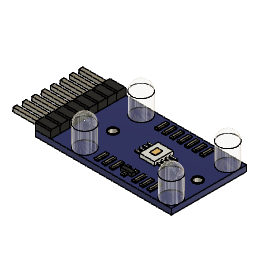
TCS3200_colour_sensor (Autodesk Fusion 360 design; units mm, degrees)
Autodesk Fusion 360 part; units mm, degrees
sketch "Circuitboard shape" plane through (0, 0, 0) normal (0, 0, 1) x (1, 0, 0)
  line L0 (0, 0) -> (36, 0)
  line L1 (36, 0) -> (36, 20)
  line L2 (36, 20) -> (0, 20)
  line L3 (0, 20) -> (0, 0)
  dimension "d1" = 20
  dimension "d2" = 36
  constraint horizontal L0
  constraint vertical L1
  constraint horizontal L2
  constraint vertical L3
  constraint coincident L0.start L3.end
  measures "d1" distance of L0.start L2.end
  measures "d2" distance of L0.start L0.end
extrude "Extrude1" add sketch "Circuitboard shape" along normal blind 1.5 makes body 1
sketch "Black Pin Connectors" plane through (0, 0, 1.5) normal (0, 0, 1) x (-1, 0, 0)
  line L0 (0, -20) -> (0, 0)
  line L1 (0, 0) -> (-36, 0)
  line L2 (-36, 0) -> (-36, -20)
  line L3 (-36, -20) -> (0, -20)
  line L4 (0, -20) -> (-4, -20)
  line L5 (-4, -20) -> (-4, -17.5)
  line L6 (-4, -17.5) -> (0, -17.5)
  line L7 (0, -17.5) -> (0, -20)
  line L8 (-4, -17.5) -> (0, -17.5)
  line L9 (0, -17.5) -> (0, -15)
  line L10 (0, -15) -> (-4, -15)
  line L11 (-4, -15) -> (-4, -17.5)
  line L12 (-4, -15) -> (0, -15)
  line L13 (0, -15) -> (0, -12.5)
  line L14 (0, -12.5) -> (-4, -12.5)
  line L15 (-4, -12.5) -> (-4, -15)
  line L16 (-4, -12.5) -> (0, -12.5)
  line L17 (0, -12.5) -> (0, -10)
  line L18 (0, -10) -> (-4, -10)
  line L19 (-4, -10) -> (-4, -12.5)
  line L20 (-4, -10) -> (0, -10)
  line L21 (0, -10) -> (0, -7.5)
  line L22 (0, -7.5) -> (-4, -7.5)
  line L23 (-4, -7.5) -> (-4, -10)
  line L24 (-4, -7.5) -> (0, -7.5)
  line L25 (0, -7.5) -> (0, -5)
  line L26 (0, -5) -> (-4, -5)
  line L27 (-4, -5) -> (-4, -7.5)
  line L28 (-4, -5) -> (0, -5)
  line L29 (0, -5) -> (0, -2.5)
  line L30 (0, -2.5) -> (-4, -2.5)
  line L31 (-4, -2.5) -> (-4, -5)
  line L32 (-4, -2.5) -> (0, -2.5)
  line L33 (0, -2.5) -> (0, 0)
  line L34 (0, 0) -> (-4, 0)
  line L35 (-4, 0) -> (-4, -2.5)
  dimension "d5" = 2.5
  dimension "d6" = 2.5
  dimension "d7" = 2.5
  dimension "d8" = 2.5
  dimension "d9" = 2.5
  dimension "d10" = 2.5
  dimension "d11" = 2.5
  dimension "d12" = 2.5
  dimension "d13" = 4
  constraint horizontal L4
  constraint vertical L5
  constraint horizontal L6
  constraint vertical L7
  constraint coincident L0.start L3.end
  constraint horizontal L8
  constraint vertical L9
  constraint horizontal L10
  constraint vertical L11
  constraint coincident L0 L9.end
  constraint horizontal L12
  constraint vertical L13
  constraint horizontal L14
  constraint vertical L15
  constraint coincident L0 L13.end
  constraint horizontal L16
  constraint vertical L17
  constraint horizontal L18
  constraint vertical L19
  constraint coincident L0 L17.end
  constraint horizontal L20
  constraint vertical L21
  constraint horizontal L22
  constraint vertical L23
  constraint coincident L0 L21.end
  constraint horizontal L24
  constraint vertical L25
  constraint horizontal L26
  constraint vertical L27
  constraint coincident L0 L25.end
  constraint horizontal L28
  constraint vertical L29
  constraint horizontal L30
  constraint vertical L31
  constraint coincident L0 L29.end
  constraint horizontal L32
  constraint vertical L33
  constraint horizontal L34
  constraint vertical L35
  constraint coincident L0.end L1.start
  measures "d5" distance of L4.end L5.end
  measures "d6" distance of L5.end L10.end
  measures "d7" distance of L10.end L14.end
  measures "d8" distance of L14.end L18.end
  measures "d9" distance of L18.end L22.end
  measures "d10" distance of L22.end L26.end
  measures "d11" distance of L26.end L30.end
  measures "d12" distance of L30.end L34.end
  measures "d13" distance of L0.end L34.end
extrude "Extrude2" add sketch "Black Pin Connectors" along normal blind 2 separate body contours L0 L3 L4 L5 L6 L7 L8 | L0 L10 L12 L13 L14 L15 L16 | L0 L18 L20 L21 L22 L23 L24 | L0 L26 L28 L29 L30 L31 L32 makes body 2 at (1.3333, 14.1667, 1.5) makes body 3 at (1.3333, 9.1667, 1.5) makes body 4 at (1.3333, 19.1667, 1.5) makes body 5 at (2.6667, 3.3333, 1.5)
chamfer "Chamfer1" distance 0.3 angle 45 8 edges at (2, 10, 3.5) (2, 7.5, 3.5) (2, 15, 3.5) (2, 12.5, 3.5) (2, 20, 3.5) (2, 17.5, 3.5) (2, 5, 3.5) (2, 2.5, 3.5) on bodies 2 3 4 5
extrude "Extrude3" add sketch "Black Pin Connectors" along normal blind 2 separate body contours L0 L6 L8 L9 L10 L11 L12 | L0 L14 L16 L17 L18 L19 L20 | L0 L1 L30 L32 L33 L34 L35 | L0 L22 L24 L25 L26 L27 L28 makes body 6 at (1.3333, 11.6667, 1.5) makes body 7 at (1.3333, 6.6667, 1.5) makes body 8 at (1.3333, 16.6667, 1.5) makes body 9 at (2.6667, 0.8333, 1.5)
chamfer "Chamfer2" distance 0.3 angle 45 8 edges at (2, 2.5, 3.5) (2, 0, 3.5) (2, 12.5, 3.5) (2, 10, 3.5) (2, 7.5, 3.5) (2, 5, 3.5) (2, 17.5, 3.5) (2, 15, 3.5) on bodies 6 7 8 9
sketch "Pins" plane through (0, 0, 0) normal (-1, 0, 0) x (0, -1, 0)
  line L0 (-17.5, 3.2) -> (-17.8, 3.5)
  line L1 (-17.8, 3.5) -> (-19.7, 3.5)
  line L2 (-19.7, 3.5) -> (-20, 3.2)
  line L3 (-20, 3.2) -> (-20, 1.5)
  line L4 (-20, 1.5) -> (-17.5, 1.5)
  line L5 (-17.5, 1.5) -> (-17.5, 3.2)
  line L6 (-15, 3.2) -> (-15.3, 3.5)
  line L7 (-15.3, 3.5) -> (-17.2, 3.5)
  line L8 (-17.2, 3.5) -> (-17.5, 3.2)
  line L9 (-17.5, 3.2) -> (-17.5, 1.5)
  line L10 (-17.5, 1.5) -> (-15, 1.5)
  line L11 (-15, 1.5) -> (-15, 3.2)
  line L12 (-12.5, 3.2) -> (-12.8, 3.5)
  line L13 (-12.8, 3.5) -> (-14.7, 3.5)
  line L14 (-14.7, 3.5) -> (-15, 3.2)
  line L15 (-15, 3.2) -> (-15, 1.5)
  line L16 (-15, 1.5) -> (-12.5, 1.5)
  line L17 (-12.5, 1.5) -> (-12.5, 3.2)
  line L18 (-10, 3.2) -> (-10.3, 3.5)
  line L19 (-10.3, 3.5) -> (-12.2, 3.5)
  line L20 (-12.2, 3.5) -> (-12.5, 3.2)
  line L21 (-12.5, 3.2) -> (-12.5, 1.5)
  line L22 (-12.5, 1.5) -> (-10, 1.5)
  line L23 (-10, 1.5) -> (-10, 3.2)
  line L24 (-7.5, 3.2) -> (-7.8, 3.5)
  line L25 (-7.8, 3.5) -> (-9.7, 3.5)
  line L26 (-9.7, 3.5) -> (-10, 3.2)
  line L27 (-10, 3.2) -> (-10, 1.5)
  line L28 (-10, 1.5) -> (-7.5, 1.5)
  line L29 (-7.5, 1.5) -> (-7.5, 3.2)
  line L30 (-5, 3.2) -> (-5.3, 3.5)
  line L31 (-5.3, 3.5) -> (-7.2, 3.5)
  line L32 (-7.2, 3.5) -> (-7.5, 3.2)
  line L33 (-7.5, 3.2) -> (-7.5, 1.5)
  line L34 (-7.5, 1.5) -> (-5, 1.5)
  line L35 (-5, 1.5) -> (-5, 3.2)
  line L36 (-2.5, 3.2) -> (-2.8, 3.5)
  line L37 (-2.8, 3.5) -> (-4.7, 3.5)
  line L38 (-4.7, 3.5) -> (-5, 3.2)
  line L39 (-5, 3.2) -> (-5, 1.5)
  line L40 (-5, 1.5) -> (-2.5, 1.5)
  line L41 (-2.5, 1.5) -> (-2.5, 3.2)
  line L42 (0, 3.2) -> (-0.3, 3.5)
  line L43 (-0.3, 3.5) -> (-2.2, 3.5)
  line L44 (-2.2, 3.5) -> (-2.5, 3.2)
  line L45 (-2.5, 3.2) -> (-2.5, 1.5)
  line L46 (-2.5, 1.5) -> (0, 1.5)
  line L47 (0, 1.5) -> (0, 3.2)
  line L48 (-19.25, 3) -> (-18.25, 3)
  line L49 (-18.25, 3) -> (-18.25, 2)
  line L50 (-18.25, 2) -> (-19.25, 2)
  line L51 (-19.25, 2) -> (-19.25, 3)
  line L52 (-16.75, 3) -> (-15.75, 3)
  line L53 (-15.75, 3) -> (-15.75, 2)
  line L54 (-15.75, 2) -> (-16.75, 2)
  line L55 (-16.75, 2) -> (-16.75, 3)
  line L56 (-14.25, 3) -> (-13.25, 3)
  line L57 (-13.25, 3) -> (-13.25, 2)
  line L58 (-13.25, 2) -> (-14.25, 2)
  line L59 (-14.25, 2) -> (-14.25, 3)
  line L60 (-11.75, 3) -> (-10.75, 3)
  line L61 (-10.75, 3) -> (-10.75, 2)
  line L62 (-10.75, 2) -> (-11.75, 2)
  line L63 (-11.75, 2) -> (-11.75, 3)
  line L64 (-9.25, 3) -> (-8.25, 3)
  line L65 (-8.25, 3) -> (-8.25, 2)
  line L66 (-8.25, 2) -> (-9.25, 2)
  line L67 (-9.25, 2) -> (-9.25, 3)
  line L68 (-6.75, 3) -> (-5.75, 3)
  line L69 (-5.75, 3) -> (-5.75, 2)
  line L70 (-5.75, 2) -> (-6.75, 2)
  line L71 (-6.75, 2) -> (-6.75, 3)
  line L72 (-4.25, 3) -> (-3.25, 3)
  line L73 (-3.25, 3) -> (-3.25, 2)
  line L74 (-3.25, 2) -> (-4.25, 2)
  line L75 (-4.25, 2) -> (-4.25, 3)
  line L76 (-1.75, 3) -> (-0.75, 3)
  line L77 (-0.75, 3) -> (-0.75, 2)
  line L78 (-0.75, 2) -> (-1.75, 2)
  line L79 (-1.75, 2) -> (-1.75, 3)
  dimension "d20" = 1
  dimension "d21" = 1
  dimension "d22" = 1
  dimension "d23" = 1
  dimension "d24" = 1
  dimension "d25" = 1
  dimension "d26" = 1
  dimension "d27" = 1
  dimension "d28" = 1
  dimension "d29" = 1
  dimension "d30" = 1
  dimension "d31" = 1
  dimension "d32" = 1
  dimension "d33" = 1
  dimension "d34" = 1
  dimension "d35" = 1
  dimension "d36" = 0.75
  dimension "d37" = 0.75
  dimension "d38" = 0.75
  dimension "d39" = 0.75
  dimension "d40" = 0.75
  dimension "d41" = 0.75
  dimension "d42" = 0.75
  dimension "d43" = 0.75
  dimension "d44" = 0.5
  dimension "d45" = 0.5
  constraint horizontal L48
  constraint vertical L49
  constraint horizontal L50
  constraint vertical L51
  constraint horizontal L52
  constraint vertical L53
  constraint horizontal L54
  constraint vertical L55
  constraint horizontal L56
  constraint vertical L57
  constraint horizontal L58
  constraint vertical L59
  constraint horizontal L60
  constraint vertical L61
  constraint horizontal L62
  constraint vertical L63
  constraint horizontal L64
  constraint vertical L65
  constraint horizontal L66
  constraint vertical L67
  constraint horizontal L68
  constraint vertical L69
  constraint horizontal L70
  constraint vertical L71
  constraint horizontal L72
  constraint vertical L73
  constraint horizontal L74
  constraint vertical L75
  constraint horizontal L76
  constraint vertical L77
  constraint horizontal L78
  constraint vertical L79
  constraint collinear L72 L76
  constraint collinear L68 L72
  constraint collinear L64 L68
  constraint collinear L60 L64
  constraint collinear L56 L60
  constraint collinear L52 L56
  constraint collinear L48 L52
  measures "d20" distance of L77.end L78.end
  measures "d21" distance of L73.end L74.end
  measures "d22" distance of L69.end L70.end
  measures "d23" distance of L65.end L66.end
  measures "d24" distance of L61.end L62.end
  measures "d25" distance of L57.end L58.end
  measures "d26" distance of L53.end L54.end
  measures "d27" distance of L49.end L50.end
  measures "d28" distance of L48.start L50.end
  measures "d29" distance of L52.start L54.end
  measures "d30" distance of L56.start L58.end
  measures "d31" distance of L60.start L62.end
  measures "d32" distance of L64.start L66.end
  measures "d33" distance of L68.start L70.end
  measures "d34" distance of L72.start L74.end
  measures "d35" distance of L76.start L78.end
  measures "d36" distance of L3 L51
  measures "d37" distance of L9 L55
  measures "d38" distance of L15 L59
  measures "d39" distance of L17 L63
  measures "d40" distance of L27 L67
  measures "d41" distance of L33 L71
  measures "d42" distance of L35 L75
  measures "d43" distance of L45 L79
  measures "d44" distance of L46 L78
  measures "d45" distance of L43 L76
extrude "Extrude4" add sketch "Pins" along normal blind 7 separate body contours L48 L49 L50 L51 | L52 L53 L54 L55 | L56 L57 L58 L59 | L60 L61 L62 L63 | L64 L65 L66 L67 | L68 L69 L70 L71 | L72 L73 L74 L75 | L76 L77 L78 L79 makes body 10 at (-2.3333, 6.4167, 3) makes body 11 at (-2.3333, 16.4167, 3) makes body 12 at (-2.3333, 13.9167, 3) makes body 13 at (-2.3333, 0.75, 2.6667) makes body 14 at (-2.3333, 8.9167, 3) makes body 15 at (-2.3333, 18.9167, 3) makes body 16 at (-2.3333, 10.75, 2.6667) makes body 17 at (-2.3333, 3.9167, 3)
fillet "Fillet1" radius 0.25 8 faces at (-7, 6.4167, 2.3333) (-7, 16.4167, 2.6667) (-7, 13.9167, 2.6667) (-7, 1.0833, 2.3333) (-7, 8.9167, 2.6667) (-7, 18.9167, 2.6667) (-7, 11.4167, 2.6667) (-7, 3.9167, 2.6667) on bodies 10 11 12 13 14 15 16 17
sketch "LEDs" plane through (0, 0, 1.5) normal (0, 0, 1) x (-1, 0, 0)
  line L0 (0, -20) -> (0, 0)
  line L1 (0, 0) -> (-36, 0)
  line L2 (-36, 0) -> (-36, -20)
  line L3 (-36, -20) -> (0, -20)
  circle A0 centre (-33.5, -17.5) radius 2.5
  circle A1 centre (-33.5, -2.5) radius 2.5
  circle A2 centre (-10.5, -17.5) radius 2.5
  circle A3 centre (-10.5, -2.5) radius 2.5
  dimension "d50" = 5
  dimension "d51" = 5
  dimension "d52" = 5
  dimension "d53" = 5
  dimension "d54" = 2.5
  dimension "d55" = 2.5
  dimension "d56" = 2.5
  dimension "d57" = 2.5
  dimension "d58" = 2.5
  dimension "d59" = 2.5
  dimension "d60" = 10.5
  dimension "d61" = 10.5
  measures "d50" diameter of A2
  measures "d51" diameter of A3
  measures "d52" diameter of A0
  measures "d53" diameter of A1
  measures "d54" distance of L3 A0.centre
  measures "d55" distance of L2 A0.centre
  measures "d56" distance of L1 A1.centre
  measures "d57" distance of L2 A1.centre
  measures "d58" distance of L1 A3.centre
  measures "d59" distance of L3 A2.centre
  measures "d60" distance of L0 A3.centre
  measures "d61" distance of L0 A2.centre
extrude "Extrude5" add sketch "LEDs" along normal blind 8 separate body contours A3 | A2 | A0 | A1 makes body 18 at (8.0124, 17.2511, 6.8333) makes body 19 at (31.0031, 2.6246, 4.1667) makes body 20 at (8.0031, 2.6246, 4.1667) makes body 21 at (31.0124, 17.2511, 6.8333)
fillet "Fillet2" radius 2.5 4 faces at (9.676, 18.5631, 9.5) (32.766, 2.6378, 9.5) (9.7813, 2.6483, 9.5) (34.2508, 16.9227, 9.5) on bodies 18 19 20 21
sketch "Colour Sensor Holder" plane through (0, 0, 1.5) normal (0, 0, 1) x (-1, 0, 0)
  line L0 (0, -20) -> (0, 0)
  line L1 (0, 0) -> (-36, 0)
  line L2 (-36, 0) -> (-36, -20)
  line L3 (-36, -20) -> (0, -20)
  line L4 (-20, -12.5) -> (-24, -12.5)
  line L5 (-24, -12.5) -> (-24, -7.5)
  line L6 (-24, -7.5) -> (-20, -7.5)
  line L7 (-20, -7.5) -> (-20, -12.5)
  dimension "d66" = 4
  dimension "d67" = 5
  dimension "d68" = 7.5
  dimension "d69" = 7.5
  dimension "d70" = 12
  constraint horizontal L4
  constraint vertical L5
  constraint horizontal L6
  constraint vertical L7
  measures "d66" distance of L5.end L6.end
  measures "d67" distance of L4.end L5.end
  measures "d68" distance of L3 L4
  measures "d69" distance of L1 L6
  measures "d70" distance of L2 L5
extrude "Extrude6" add sketch "Colour Sensor Holder" along normal blind 1 separate body contours L4 L5 L6 L7 makes body 22
sketch "Colour Sensor Matrix" plane through (0, 0, 2.5) normal (0, 0, 1) x (-1, 0, 0)
  line L0 (-20, -7.5) -> (-24, -7.5)
  line L1 (-24, -7.5) -> (-24, -12.5)
  line L2 (-24, -12.5) -> (-20, -12.5)
  line L3 (-20, -12.5) -> (-20, -7.5)
  line L4 (-21.25, -11) -> (-22.75, -11)
  line L5 (-22.75, -11) -> (-22.75, -9)
  line L6 (-22.75, -9) -> (-21.25, -9)
  line L7 (-21.25, -9) -> (-21.25, -11)
  dimension "d73" = 1.5
  dimension "d74" = 2
  dimension "d75" = 5
  dimension "d76" = 1.5
  dimension "d77" = 1.5
  dimension "d78" = 4
  dimension "d79" = 1.25
  dimension "d80" = 1.25
  constraint horizontal L4
  constraint vertical L5
  constraint horizontal L6
  constraint vertical L7
  measures "d73" distance of L5.end L6.end
  measures "d74" distance of L4.end L5.end
  measures "d75" distance of L0 L2
  measures "d76" distance of L2 L4
  measures "d77" distance of L0 L6
  measures "d78" distance of L1 L3
  measures "d79" distance of L3 L7
  measures "d80" distance of L1 L5
extrude "Extrude7" add sketch "Colour Sensor Matrix" along normal blind 0.1 separate body contours L4 L5 L6 L7 makes body 23
sketch "Surface Components" plane through (0, 0, 1.5) normal (0, 0, 1) x (-1, 0, 0)
  line L0 (0, -20) -> (0, 0)
  line L1 (0, 0) -> (-36, 0)
  line L2 (-36, 0) -> (-36, -20)
  line L3 (-36, -20) -> (0, -20)
  line L4 (-28.5, -19) -> (-27.5, -19)
  line L5 (-27.5, -19) -> (-27.5, -16)
  line L6 (-27.5, -16) -> (-28.5, -16)
  line L7 (-28.5, -16) -> (-28.5, -19)
  line L8 (-26.5, -19) -> (-25.5, -19)
  line L9 (-25.5, -19) -> (-25.5, -16)
  line L10 (-25.5, -16) -> (-26.5, -16)
  line L11 (-26.5, -16) -> (-26.5, -19)
  line L12 (-24.5, -19) -> (-23.5, -19)
  line L13 (-23.5, -19) -> (-23.5, -16)
  line L14 (-23.5, -16) -> (-24.5, -16)
  line L15 (-24.5, -16) -> (-24.5, -19)
  line L16 (-22.5, -19) -> (-21.5, -19)
  line L17 (-21.5, -19) -> (-21.5, -16)
  line L18 (-21.5, -16) -> (-22.5, -16)
  line L19 (-22.5, -16) -> (-22.5, -19)
  line L20 (-20.5, -19) -> (-19.5, -19)
  line L21 (-19.5, -19) -> (-19.5, -16)
  line L22 (-19.5, -16) -> (-20.5, -16)
  line L23 (-20.5, -16) -> (-20.5, -19)
  line L24 (-18.5, -19) -> (-17.5, -19)
  line L25 (-17.5, -19) -> (-17.5, -16)
  line L26 (-17.5, -16) -> (-18.5, -16)
  line L27 (-18.5, -16) -> (-18.5, -19)
  line L28 (-16.5, -19) -> (-15.5, -19)
  line L29 (-15.5, -19) -> (-15.5, -16)
  line L30 (-15.5, -16) -> (-16.5, -16)
  line L31 (-16.5, -16) -> (-16.5, -19)
  line L32 (-14.5, -1) -> (-15.5, -1)
  line L33 (-15.5, -1) -> (-15.5, -4)
  line L34 (-15.5, -4) -> (-14.5, -4)
  line L35 (-14.5, -4) -> (-14.5, -1)
  line L36 (-16.5, -1) -> (-17.5, -1)
  line L37 (-17.5, -1) -> (-17.5, -4)
  line L38 (-17.5, -4) -> (-16.5, -4)
  line L39 (-16.5, -4) -> (-16.5, -1)
  line L40 (-18.5, -1) -> (-19.5, -1)
  line L41 (-19.5, -1) -> (-19.5, -4)
  line L42 (-19.5, -4) -> (-18.5, -4)
  line L43 (-18.5, -4) -> (-18.5, -1)
  line L44 (-29.5, -1) -> (-28.5, -1)
  line L45 (-28.5, -1) -> (-28.5, -4)
  line L46 (-28.5, -4) -> (-29.5, -4)
  line L47 (-29.5, -4) -> (-29.5, -1)
  line L48 (-27.5, -1) -> (-26.5, -1)
  line L49 (-26.5, -1) -> (-26.5, -4)
  line L50 (-26.5, -4) -> (-27.5, -4)
  line L51 (-27.5, -4) -> (-27.5, -1)
  line L52 (-25.5, -1) -> (-24.5, -1)
  line L53 (-24.5, -1) -> (-24.5, -4)
  line L54 (-24.5, -4) -> (-25.5, -4)
  line L55 (-25.5, -4) -> (-25.5, -1)
  line L56 (-20.5, -3) -> (-23.5, -3)
  line L57 (-23.5, -3) -> (-23.5, -2)
  line L58 (-23.5, -2) -> (-20.5, -2)
  line L59 (-20.5, -2) -> (-20.5, -3)
  line L60 (-21.5, -2) -> (-22.5, -2)
  line L61 (-22.5, -2) -> (-22.5, -1)
  line L62 (-22.5, -1) -> (-21.5, -1)
  line L63 (-21.5, -1) -> (-21.5, -2)
  line L64 (-20.5, -3) -> (-21.5, -3)
  line L65 (-21.5, -3) -> (-21.5, -4)
  line L66 (-21.5, -4) -> (-20.5, -4)
  line L67 (-20.5, -4) -> (-20.5, -3)
  line L68 (-22.5, -3) -> (-23.5, -3)
  line L69 (-23.5, -3) -> (-23.5, -4)
  line L70 (-23.5, -4) -> (-22.5, -4)
  line L71 (-22.5, -4) -> (-22.5, -3)
  dimension "d84" = 1
  dimension "d85" = 1
  dimension "d86" = 1
  dimension "d87" = 1
  dimension "d88" = 1
  dimension "d89" = 1
  dimension "d90" = 1
  dimension "d91" = 1
  dimension "d92" = 1
  dimension "d93" = 1
  dimension "d94" = 1
  dimension "d95" = 1
  dimension "d96" = 1
  dimension "d98" = 7.5
  dimension "d99" = 3
  dimension "d100" = 1
  dimension "d101" = 1
  dimension "d102" = 1
  dimension "d103" = 1
  dimension "d104" = 1
  dimension "d105" = 1
  dimension "d106" = 1
  dimension "d107" = 1
  dimension "d108" = 3
  dimension "d109" = 1
  dimension "d110" = 1
  dimension "d111" = 1
  dimension "d112" = 1
  dimension "d113" = 6.5
  dimension "d114" = 1
  dimension "d115" = 1
  dimension "d116" = 3
  dimension "d117" = 1
  dimension "d118" = 2
  dimension "d119" = 1
  dimension "d120" = 1
  dimension "d121" = 1
  dimension "d122" = 1
  dimension "d123" = 1
  constraint horizontal L4
  constraint vertical L5
  constraint horizontal L6
  constraint vertical L7
  constraint horizontal L8
  constraint vertical L9
  constraint horizontal L10
  constraint vertical L11
  constraint horizontal L12
  constraint vertical L13
  constraint horizontal L14
  constraint vertical L15
  constraint horizontal L16
  constraint vertical L17
  constraint horizontal L18
  constraint vertical L19
  constraint horizontal L20
  constraint vertical L21
  constraint horizontal L22
  constraint vertical L23
  constraint horizontal L24
  constraint vertical L25
  constraint horizontal L26
  constraint vertical L27
  constraint horizontal L28
  constraint vertical L29
  constraint horizontal L30
  constraint vertical L31
  constraint collinear L6 L10
  constraint collinear L10 L14
  constraint collinear L14 L18
  constraint collinear L18 L22
  constraint collinear L22 L26
  constraint collinear L26 L30
  constraint collinear L4 L8
  constraint collinear L8 L12
  constraint collinear L12 L16
  constraint collinear L16 L20
  constraint collinear L20 L24
  constraint collinear L24 L28
  constraint horizontal L32
  constraint vertical L33
  constraint horizontal L34
  constraint vertical L35
  constraint horizontal L36
  constraint vertical L37
  constraint horizontal L38
  constraint vertical L39
  constraint horizontal L40
  constraint vertical L41
  constraint horizontal L42
  constraint vertical L43
  constraint horizontal L44
  constraint vertical L45
  constraint horizontal L46
  constraint vertical L47
  constraint horizontal L48
  constraint vertical L49
  constraint horizontal L50
  constraint vertical L51
  constraint horizontal L52
  constraint vertical L53
  constraint horizontal L54
  constraint vertical L55
  constraint horizontal L56
  constraint vertical L57
  constraint horizontal L58
  constraint vertical L59
  constraint horizontal L60
  constraint vertical L61
  constraint horizontal L62
  constraint vertical L63
  constraint coincident L58 L60.start
  constraint horizontal L64
  constraint vertical L65
  constraint horizontal L66
  constraint vertical L67
  constraint coincident L56 L59.end
  constraint horizontal L68
  constraint vertical L69
  constraint horizontal L70
  constraint vertical L71
  constraint coincident L56 L68.start
  constraint collinear L44 L48
  constraint collinear L48 L52
  constraint collinear L40 L52
  constraint collinear L36 L40
  constraint collinear L32 L36
  constraint collinear L46 L50
  constraint collinear L50 L54
  constraint collinear L42 L54
  constraint collinear L38 L42
  constraint collinear L34 L38
  constraint collinear L59 L67
  constraint collinear L57 L69
  constraint collinear L54 L70
  constraint collinear L42 L66
  constraint collinear L52 L62
  measures "d84" distance of L4.start L4.end
  measures "d85" distance of L8.start L8.end
  measures "d86" distance of L12.start L12.end
  measures "d87" distance of L16.start L16.end
  measures "d88" distance of L20.start L20.end
  measures "d89" distance of L24.start L24.end
  measures "d90" distance of L28.start L28.end
  measures "d91" distance of L25 L31
  measures "d92" distance of L21 L27
  measures "d93" distance of L17 L23
  measures "d94" distance of L13 L19
  measures "d95" distance of L9 L15
  measures "d96" distance of L5 L11
  measures "d98" distance of L2 L7
  measures "d99" distance of L4.start L6.end
  measures "d100" distance of L3 L4
  measures "d101" distance of L32.start L32.end
  measures "d102" distance of L36.start L36.end
  measures "d103" distance of L40.start L40.end
  measures "d104" distance of L52.start L52.end
  measures "d105" distance of L48.start L48.end
  measures "d106" distance of L44.start L44.end
  measures "d107" distance of L1 L44
  measures "d108" distance of L44.start L46.end
  measures "d109" distance of L33 L39
  measures "d110" distance of L37 L43
  measures "d111" distance of L49 L55
  measures "d112" distance of L45 L51
  measures "d113" distance of L2 L47
  measures "d114" distance of L41 L59
  measures "d115" distance of L53 L57
  measures "d116" distance of L57.end L58.end
  measures "d117" distance of L56.start L58.end
  measures "d118" distance of L1 L58
  measures "d119" distance of L69.end L70.end
  measures "d120" distance of L65.end L66.end
  measures "d121" distance of L61.end L62.end
  measures "d122" distance of L57 L61
  measures "d123" distance of L59 L63
extrude "Extrude8" add sketch "Surface Components" along normal blind 0.5 separate body contours L4 L5 L6 L7 | L8 L9 L10 L11 | L12 L13 L14 L15 | L16 L17 L18 L19 | L20 L21 L22 L23 | L24 L25 L26 L27 | L28 L29 L30 L31 | L32 L33 L34 L35 | L36 L37 L38 L39 | L40 L41 L42 L43 | L44 L45 L46 L47 | L48 L49 L50 L51 | L52 L53 L54 L55 | L56 L64 L65 L66 L67 | L56 L68 L69 L70 L71 | L58 L60 L61 L62 L63 makes body 24 at (25.1667, 2, 1.5) makes body 25 at (19.1667, 2, 1.5) makes body 26 at (26.1667, 17, 1.5) makes body 27 at (18.1667, 17, 1.5) makes body 28 at (20.1667, 17, 1.5) makes body 29 at (28.1667, 17, 1.5) makes body 30 at (21.1667, 3.3333, 1.5) makes body 31 at (27.1667, 2, 1.5) makes body 32 at (22.1667, 1.3333, 1.5) makes body 33 at (17.1667, 3, 1.5) makes body 34 at (24.1667, 17, 1.5) makes body 35 at (16.1667, 17, 1.5) makes body 36 at (22.1667, 17, 1.5) makes body 37 at (15.1667, 2, 1.5) makes body 38 at (22.8333, 3.6667, 1.5) makes body 39 at (29.1667, 2, 1.5)
extrude "Extrude9" add sketch "Surface Components" along normal blind 0.8 separate body contours L56 L57 L58 L59 L60 L64 L68 makes body 40
fillet "Fillet3" radius 0.2 16 faces at (25.1667, 2, 2) (19.1667, 2, 2) (26.1667, 17, 2) (18.1667, 17, 2) (20.1667, 17, 2) (28.1667, 17, 2) (21.1667, 3.3333, 2) (27.1667, 2, 2) (22.1667, 1.3333, 2) (17.1667, 3, 2) (24.1667, 17, 2) (16.1667, 17, 2) (22.1667, 17, 2) (15.1667, 2, 2) (22.8333, 3.6667, 2) (29.1667, 2, 2) on bodies 24 25 26 27 28 29 30 31 32 33 34 35 36 37 38 39
sketch "Holes" plane through (0, 0, 1.5) normal (0, 0, 1) x (-1, 0, 0)
  line L0 (0, -20) -> (0, 0)
  line L1 (0, 0) -> (-36, 0)
  line L2 (-36, 0) -> (-36, -20)
  line L3 (-36, -20) -> (0, -20)
  circle A0 centre (-33, -10) radius 1
  circle A1 centre (-10.5, -10) radius 1
  circle A2 centre (-10.5, -10) radius 1.25
  circle A3 centre (-33, -10) radius 1.25
  dimension "d130" = 2
  dimension "d131" = 2
  dimension "d132" = 3
  dimension "d133" = 10.5
  dimension "d134" = 10
  dimension "d135" = 10
  dimension "d136" = 2.5
  dimension "d137" = 2.5
  constraint concentric A1 A2
  constraint concentric A0 A3
  measures "d130" diameter of A1
  measures "d131" diameter of A0
  measures "d132" distance of L2 A0.centre
  measures "d133" distance of L0 A1.centre
  measures "d134" distance of L3 A0.centre
  measures "d135" distance of L3 A1.centre
  measures "d136" diameter of A2
  measures "d137" diameter of A3
extrude "Extrude10" cut sketch "Holes" against normal blind 1.5 contours A0 | A1 bodies 1
extrude "Extrude11" add sketch "Holes" along normal blind 0.2 separate body contours A2 | A3 makes body 41 at (9.338, 10.0621, 1.5) makes body 42 at (31.838, 10.0621, 1.5)
sketch "Bottom Holes" plane through (0, 0, 0) normal (0, 0, -1) x (1, 0, 0)
  circle A0 centre (10.5, -10) radius 1
  circle A1 centre (33, -10) radius 1
  line L0 (0, 0) -> (0, -20)
  line L1 (0, -20) -> (36, -20)
  line L2 (36, -20) -> (36, 0)
  line L3 (36, 0) -> (0, 0)
  circle A2 centre (10.5, -10) radius 1
  circle A3 centre (33, -10) radius 1
  circle A4 centre (10.5, -10) radius 1.25
  circle A5 centre (33, -10) radius 1.25
  dimension "d142" = 2.5
  dimension "d143" = 2.5
  constraint concentric A2 A4
  constraint concentric A3 A5
  measures "d142" diameter of A4
  measures "d143" diameter of A5
extrude "Extrude12" add sketch "Bottom Holes" along normal blind 0.2 separate body contours A4 | A5 makes body 43 at (11.662, 10.0621, 0) makes body 44 at (33.5272, 11.0374, 0)
fillet "Fillet4" radius 0.1 4 faces at (9.338, 10.0621, 1.7) (31.838, 10.0621, 1.7) (11.662, 10.0621, -0.2) (33.5272, 11.0374, -0.2) on bodies 41 42 43 44
sketch "Bottom Pins" plane through (0, 0, 0) normal (0, 0, -1) x (1, 0, 0)
  circle A0 centre (10.5, -10) radius 1
  circle A1 centre (33, -10) radius 1
  line L0 (0, 0) -> (0, -20)
  line L1 (0, -20) -> (36, -20)
  line L2 (36, -20) -> (36, 0)
  line L3 (36, 0) -> (0, 0)
  line L4 (4, -17.5) -> (0, -17.5)
  line L5 (0, -20) -> (4, -20)
  line L6 (0, -15) -> (4, -15)
  line L7 (0, -12.5) -> (4, -12.5)
  line L8 (4, -10) -> (0, -10)
  line L9 (4, -7.5) -> (0, -7.5)
  line L10 (4, -5) -> (0, -5)
  line L11 (4, -2.5) -> (0, -2.5)
  line L12 (0, 0) -> (4, 0)
  line L13 (4, 0) -> (4, -2.5)
  line L14 (0, -2.5) -> (0, 0)
  line L15 (0, -5) -> (0, -2.5)
  line L16 (4, -2.5) -> (4, -5)
  line L17 (0, -7.5) -> (0, -5)
  line L18 (4, -5) -> (4, -7.5)
  line L19 (4, -7.5) -> (4, -10)
  line L20 (0, -10) -> (0, -7.5)
  line L21 (0, -12.5) -> (0, -10)
  line L22 (0, -15) -> (0, -12.5)
  line L23 (0, -17.5) -> (0, -15)
  line L24 (0, -17.5) -> (0, -20)
  line L25 (4, -20) -> (4, -17.5)
  line L26 (4, -15) -> (4, -17.5)
  line L27 (4, -12.5) -> (4, -15)
  line L28 (4, -10) -> (4, -12.5)
  line L29 (2, -0.75) -> (3, -0.75)
  line L30 (3, -0.75) -> (3, -1.75)
  line L31 (3, -1.75) -> (2, -1.75)
  line L32 (2, -1.75) -> (2, -0.75)
  line L33 (2, -3.25) -> (3, -3.25)
  line L34 (3, -3.25) -> (3, -4.25)
  line L35 (3, -4.25) -> (2, -4.25)
  line L36 (2, -4.25) -> (2, -3.25)
  line L37 (2, -5.75) -> (3, -5.75)
  line L38 (3, -5.75) -> (3, -6.75)
  line L39 (3, -6.75) -> (2, -6.75)
  line L40 (2, -6.75) -> (2, -5.75)
  line L41 (2, -8.25) -> (3, -8.25)
  line L42 (3, -8.25) -> (3, -9.25)
  line L43 (3, -9.25) -> (2, -9.25)
  line L44 (2, -9.25) -> (2, -8.25)
  line L45 (2, -10.75) -> (3, -10.75)
  line L46 (3, -10.75) -> (3, -11.75)
  line L47 (3, -11.75) -> (2, -11.75)
  line L48 (2, -11.75) -> (2, -10.75)
  line L49 (2, -13.25) -> (3, -13.25)
  line L50 (3, -13.25) -> (3, -14.25)
  line L51 (3, -14.25) -> (2, -14.25)
  line L52 (2, -14.25) -> (2, -13.25)
  line L53 (2, -15.75) -> (3, -15.75)
  line L54 (3, -15.75) -> (3, -16.75)
  line L55 (3, -16.75) -> (2, -16.75)
  line L56 (2, -16.75) -> (2, -15.75)
  line L57 (2, -18.25) -> (3, -18.25)
  line L58 (3, -18.25) -> (3, -19.25)
  line L59 (3, -19.25) -> (2, -19.25)
  line L60 (2, -19.25) -> (2, -18.25)
  line L61 (4, -15) -> (0, -15)
  line L62 (4, -17.5) -> (0, -17.5)
  line L63 (35, -2) -> (33, -2)
  line L64 (33, -2) -> (33, -4)
  line L65 (33, -4) -> (35, -4)
  line L66 (35, -4) -> (35, -2)
  line L67 (32, -2) -> (30, -2)
  line L68 (30, -2) -> (30, -4)
  line L69 (30, -4) -> (32, -4)
  line L70 (32, -4) -> (32, -2)
  line L71 (8, -2) -> (10, -2)
  line L72 (10, -2) -> (10, -4)
  line L73 (10, -4) -> (8, -4)
  line L74 (8, -4) -> (8, -2)
  line L75 (11, -2) -> (13, -2)
  line L76 (13, -2) -> (13, -4)
  line L77 (13, -4) -> (11, -4)
  line L78 (11, -4) -> (11, -2)
  line L79 (35, -16) -> (33, -16)
  line L80 (33, -16) -> (33, -18)
  line L81 (33, -18) -> (35, -18)
  line L82 (35, -18) -> (35, -16)
  line L83 (32, -16) -> (30, -16)
  line L84 (30, -16) -> (30, -18)
  line L85 (30, -18) -> (32, -18)
  line L86 (32, -18) -> (32, -16)
  line L87 (13, -16) -> (11, -16)
  line L88 (11, -16) -> (11, -18)
  line L89 (11, -18) -> (13, -18)
  line L90 (13, -18) -> (13, -16)
  line L91 (10, -16) -> (8, -16)
  line L92 (8, -16) -> (8, -18)
  line L93 (8, -18) -> (10, -18)
  line L94 (10, -18) -> (10, -16)
  dimension "d148" = 1
  dimension "d149" = 0.75
  dimension "d150" = 0.75
  dimension "d151" = 0.75
  dimension "d152" = 0.75
  dimension "d153" = 0.75
  dimension "d154" = 0.75
  dimension "d155" = 0.75
  dimension "d156" = 0.75
  dimension "d157" = 1
  dimension "d158" = 1
  dimension "d159" = 1
  dimension "d160" = 1
  dimension "d161" = 1
  dimension "d162" = 1
  dimension "d163" = 1
  dimension "d164" = 1
  dimension "d165" = 2
  dimension "d167" = 2
  dimension "d168" = 2
  dimension "d169" = 2
  dimension "d170" = 2
  dimension "d171" = 2
  dimension "d172" = 2
  dimension "d173" = 2
  dimension "d174" = 2
  dimension "d175" = 1
  dimension "d176" = 1
  dimension "d177" = 1
  dimension "d178" = 8
  constraint horizontal L29
  constraint vertical L30
  constraint horizontal L31
  constraint vertical L32
  constraint horizontal L33
  constraint vertical L34
  constraint horizontal L35
  constraint vertical L36
  constraint horizontal L37
  constraint vertical L38
  constraint horizontal L39
  constraint vertical L40
  constraint horizontal L41
  constraint vertical L42
  constraint horizontal L43
  constraint vertical L44
  constraint horizontal L45
  constraint vertical L46
  constraint horizontal L47
  constraint vertical L48
  constraint horizontal L49
  constraint vertical L50
  constraint horizontal L51
  constraint vertical L52
  constraint horizontal L53
  constraint vertical L54
  constraint horizontal L55
  constraint vertical L56
  constraint horizontal L57
  constraint vertical L58
  constraint horizontal L59
  constraint vertical L60
  constraint collinear L54 L58
  constraint collinear L50 L54
  constraint collinear L46 L50
  constraint collinear L42 L46
  constraint collinear L38 L42
  constraint collinear L34 L38
  constraint collinear L30 L34
  constraint collinear L32 L36
  constraint collinear L36 L40
  constraint collinear L40 L44
  constraint collinear L44 L48
  constraint collinear L48 L52
  constraint collinear L52 L56
  constraint collinear L56 L60
  constraint horizontal L63
  constraint vertical L64
  constraint horizontal L65
  constraint vertical L66
  constraint horizontal L67
  constraint vertical L68
  constraint horizontal L69
  constraint vertical L70
  constraint horizontal L71
  constraint vertical L72
  constraint horizontal L73
  constraint vertical L74
  constraint horizontal L75
  constraint vertical L76
  constraint horizontal L77
  constraint vertical L78
  constraint collinear L63 L67
  constraint collinear L67 L75
  constraint collinear L71 L75
  constraint collinear L73 L77
  constraint collinear L69 L77
  constraint collinear L65 L69
  constraint horizontal L79
  constraint vertical L80
  constraint horizontal L81
  constraint vertical L82
  constraint horizontal L83
  constraint vertical L84
  constraint horizontal L85
  constraint vertical L86
  constraint horizontal L87
  constraint vertical L88
  constraint horizontal L89
  constraint vertical L90
  constraint horizontal L91
  constraint vertical L92
  constraint horizontal L93
  constraint vertical L94
  constraint collinear L87 L91
  constraint collinear L83 L87
  constraint collinear L79 L83
  constraint collinear L81 L85
  constraint collinear L85 L89
  constraint collinear L89 L93
  constraint collinear L66 L82
  constraint collinear L64 L80
  constraint collinear L70 L86
  constraint collinear L68 L84
  constraint collinear L74 L92
  constraint collinear L72 L94
  constraint collinear L78 L88
  constraint collinear L76 L90
  measures "d148" distance of L58.end L59.end
  measures "d149" distance of L12 L29
  measures "d150" distance of L11 L33
  measures "d151" distance of L10 L37
  measures "d152" distance of L9 L41
  measures "d153" distance of L8 L45
  measures "d154" distance of L7 L49
  measures "d155" distance of L53 L61
  measures "d156" distance of L57 L62
  measures "d157" distance of L57.end L58.end
  measures "d158" distance of L53.end L54.end
  measures "d159" distance of L49.end L50.end
  measures "d160" distance of L45.end L46.end
  measures "d161" distance of L41.end L42.end
  measures "d162" distance of L37.end L38.end
  measures "d163" distance of L33.end L34.end
  measures "d164" distance of L29.end L30.end
  measures "d165" distance of L24 L60
  measures "d167" distance of L63.start L65.end
  measures "d168" distance of L3 L63
  measures "d169" distance of L79.start L81.end
  measures "d170" distance of L1 L81
  measures "d171" distance of L80.end L81.end
  measures "d172" distance of L84.end L85.end
  measures "d173" distance of L88.end L89.end
  measures "d174" distance of L92.end L93.end
  measures "d175" distance of L2 L82
  measures "d176" distance of L80 L86
  measures "d177" distance of L88 L94
  measures "d178" distance of L23 L92
extrude "Extrude13" add sketch "Bottom Pins" along normal blind 1 separate body contours L29 L30 L31 L32 | L33 L34 L35 L36 | L37 L38 L39 L40 | L41 L42 L43 L44 | L45 L46 L47 L48 | L49 L50 L51 L52 | L53 L54 L55 L56 | L57 L58 L59 L60 | L63 L64 L65 L66 | L67 L68 L69 L70 | L71 L72 L73 L74 | L75 L76 L77 L78 | L79 L80 L81 L82 | L83 L84 L85 L86 | L87 L88 L89 L90 | L91 L92 L93 L94 makes body 45 at (34.3333, 3.3333, 0) makes body 46 at (11.6667, 2.6667, 0) makes body 47 at (2.3333, 13.25, -0.3333) makes body 48 at (2.3333, 3.25, -0.3333) makes body 49 at (2.3333, 5.75, -0.3333) makes body 50 at (3, 16.0833, -0.3333) makes body 51 at (8.6667, 16.6667, 0) makes body 52 at (30.6667, 16.6667, 0) makes body 53 at (31.3333, 3.3333, 0) makes body 54 at (8.6667, 2.6667, 0) makes body 55 at (2.3333, 10.75, -0.3333) makes body 56 at (2.3333, 0.75, -0.3333) makes body 57 at (2.3333, 8.25, -0.3333) makes body 58 at (2.3333, 18.25, -0.3333) makes body 59 at (11.6667, 16.6667, 0) makes body 60 at (33.6667, 17.3333, 0)
chamfer "Chamfer3" distance 0.4 angle 45 8 faces at (2.3333, 8.5833, -1) (2.3333, 11.0833, -1) (2.3333, 16.0833, -1) (2.3333, 3.5833, -1) (2.6667, 6.4167, -1) (2.3333, 13.5833, -1) (2.3333, 1.0833, -1) (2.3333, 18.5833, -1) on bodies 47 48 49 50 55 56 57 58
chamfer "Chamfer4" distance 0.9 angle 45 8 faces at (8.6667, 2.6667, -1) (11.6667, 2.6667, -1) (34.3333, 3.3333, -1) (31.3333, 3.3333, -1) (30.6667, 16.6667, -1) (8.6667, 16.6667, -1) (11.6667, 16.6667, -1) (33.6667, 17.3333, -1) on bodies 45 46 51 52 53 54 59 60
sketch "Sketch13" plane through (0, 0, 1.5) normal (0, 0, 1) x (-1, 0, 0)
  circle A0 centre (-10.5, -10) radius 1
  circle A1 centre (-33, -10) radius 1
  line L0 (0, -20) -> (0, 0)
  line L1 (0, 0) -> (-36, 0)
  line L2 (-36, 0) -> (-36, -20)
  line L3 (-36, -20) -> (0, -20)
  line L4 (-20, -7.5) -> (-24, -7.5)
  line L5 (-24, -7.5) -> (-24, -12.5)
  line L6 (-24, -12.5) -> (-20, -12.5)
  line L7 (-20, -12.5) -> (-20, -7.5)
  line L8 (-24, -11.82) -> (-26, -11.82)
  line L9 (-26, -11.82) -> (-26, -11.42)
  line L10 (-26, -11.42) -> (-24, -11.42)
  line L11 (-24, -11.42) -> (-24, -11.82)
  line L12 (-24, -10.74) -> (-26, -10.74)
  line L13 (-26, -10.74) -> (-26, -10.34)
  line L14 (-26, -10.34) -> (-24, -10.34)
  line L15 (-24, -10.34) -> (-24, -10.74)
  line L16 (-24, -9.66) -> (-26, -9.66)
  line L17 (-26, -9.66) -> (-26, -9.26)
  line L18 (-26, -9.26) -> (-24, -9.26)
  line L19 (-24, -9.26) -> (-24, -9.66)
  line L20 (-24, -8.58) -> (-26, -8.58)
  line L21 (-26, -8.58) -> (-26, -8.18)
  line L22 (-26, -8.18) -> (-24, -8.18)
  line L23 (-24, -8.18) -> (-24, -8.58)
  line L24 (-20, -11.82) -> (-18, -11.82)
  line L25 (-18, -11.82) -> (-18, -11.42)
  line L26 (-18, -11.42) -> (-20, -11.42)
  line L27 (-20, -11.42) -> (-20, -11.82)
  line L28 (-20, -10.74) -> (-18, -10.74)
  line L29 (-18, -10.74) -> (-18, -10.34)
  line L30 (-18, -10.34) -> (-20, -10.34)
  line L31 (-20, -10.34) -> (-20, -10.74)
  line L32 (-20, -9.66) -> (-18, -9.66)
  line L33 (-18, -9.66) -> (-18, -9.26)
  line L34 (-18, -9.26) -> (-20, -9.26)
  line L35 (-20, -9.26) -> (-20, -9.66)
  line L36 (-20, -8.58) -> (-18, -8.58)
  line L37 (-18, -8.58) -> (-18, -8.18)
  line L38 (-18, -8.18) -> (-20, -8.18)
  line L39 (-20, -8.18) -> (-20, -8.58)
  dimension "d189" = 0.4
  dimension "d190" = 0.4
  dimension "d191" = 0.4
  dimension "d192" = 0.4
  dimension "d193" = 2
  dimension "d194" = 2
  dimension "d195" = 0.68
  dimension "d196" = 0.68
  dimension "d197" = 0.68
  dimension "d198" = 0.68
  dimension "d199" = 0.68
  dimension "d200" = 0.68
  constraint horizontal L8
  constraint vertical L9
  constraint horizontal L10
  constraint vertical L11
  constraint coincident L5 L8.start
  constraint horizontal L12
  constraint vertical L13
  constraint horizontal L14
  constraint vertical L15
  constraint coincident L5 L12.start
  constraint horizontal L16
  constraint vertical L17
  constraint horizontal L18
  constraint vertical L19
  constraint coincident L5 L16.start
  constraint horizontal L20
  constraint vertical L21
  constraint horizontal L22
  constraint vertical L23
  constraint coincident L5 L20.start
  constraint horizontal L24
  constraint vertical L25
  constraint horizontal L26
  constraint vertical L27
  constraint coincident L7 L24.start
  constraint horizontal L28
  constraint vertical L29
  constraint horizontal L30
  constraint vertical L31
  constraint coincident L7 L28.start
  constraint horizontal L32
  constraint vertical L33
  constraint horizontal L34
  constraint vertical L35
  constraint coincident L7 L32.start
  constraint horizontal L36
  constraint vertical L37
  constraint horizontal L38
  constraint vertical L39
  constraint coincident L7 L36.start
  constraint collinear L9 L13
  constraint collinear L17 L21
  constraint collinear L13 L17
  constraint collinear L25 L29
  constraint collinear L29 L33
  constraint collinear L33 L37
  constraint collinear L8 L24
  constraint collinear L12 L28
  constraint collinear L16 L32
  constraint collinear L20 L36
  constraint collinear L10 L26
  constraint collinear L14 L30
  constraint collinear L18 L34
  constraint collinear L22 L38
  measures "d189" distance of L8.end L9.end
  measures "d190" distance of L12.end L13.end
  measures "d191" distance of L16.end L17.end
  measures "d192" distance of L20.end L21.end
  measures "d193" distance of L21.end L22.end
  measures "d194" distance of L37.end L38.end
  measures "d195" distance of L6 L8
  measures "d196" distance of L10 L12
  measures "d197" distance of L14 L16
  measures "d198" distance of L18 L20
  measures "d199" distance of L4 L22
  measures "d200" distance of L6 L24
extrude "Extrude14" add sketch "Sketch13" along normal blind 0.5 separate body contours L7 L36 L37 L38 L39 | L5 L20 L21 L22 L23 | L7 L32 L33 L34 L35 | L5 L16 L17 L18 L19 | L7 L28 L29 L30 L31 | L5 L12 L13 L14 L15 | L7 L24 L25 L26 L27 | L5 L8 L9 L10 L11 makes body 61 at (25.3333, 10.34, 1.6667) makes body 62 at (18.6667, 10.34, 1.6667) makes body 63 at (18.6667, 9.26, 1.6667) makes body 64 at (25.3333, 9.26, 1.6667) makes body 65 at (25.3333, 11.42, 1.6667) makes body 66 at (18.6667, 11.42, 1.6667) makes body 67 at (18.6667, 8.18, 1.6667) makes body 68 at (25.3333, 8.18, 1.6667)
fillet "Fillet8" radius 0.2 40 edges at (25, 10.34, 2) (25, 10.74, 2) (26, 10.54, 2) (26, 10.34, 1.75) (26, 10.74, 1.75) (19, 10.74, 2) (19, 10.34, 2) (18, 10.54, 2) (18, 10.74, 1.75) (18, 10.34, 1.75) (18, 9.66, 1.75) (18, 9.46, 2) (18, 9.26, 1.75) (19, 9.26, 2) (19, 9.66, 2) (25, 9.26, 2) (25, 9.66, 2) (26, 9.46, 2) (26, 9.26, 1.75) (26, 9.66, 1.75) (25, 11.42, 2) (25, 11.82, 2) (26, 11.62, 2) (26, 11.42, 1.75) (26, 11.82, 1.75) (19, 11.82, 2) (19, 11.42, 2) (18, 11.62, 2) (18, 11.82, 1.75) (18, 11.42, 1.75) (18, 8.18, 1.75) (18, 8.58, 1.75) (19, 8.58, 2) (18, 8.38, 2) (19, 8.18, 2) (25, 8.18, 2) (25, 8.58, 2) (26, 8.38, 2) (26, 8.18, 1.75) (26, 8.58, 1.75) on bodies 61 62 63 64 65 66 67 68
equation "d5 = ( 20 / 8 ) * 1 mm"
equation "d6 = ( 20 / 8 ) * 1 mm"
equation "d7 = ( 20 / 8 ) * 1 mm"
equation "d8 = ( 20 / 8 ) * 1 mm"
equation "d9 = ( 20 / 8 ) * 1 mm"
equation "d10 = ( 20 / 8 ) * 1 mm"
equation "d11 = ( 20 / 8 ) * 1 mm"
equation "d36 = ( ( 2.5 - 1 ) / 2 ) * 1 mm"
equation "d68 = ( ( 20 - 5 ) / 2 ) * 1 mm"
equation "d76 = ( ( 5 - 2 ) / 2 ) * 1 mm"
equation "d79 = ( ( 4 - 1.5 ) / 2 ) * 1 mm"
equation "d195 = ( ( 5 - 4 * 0.4 ) / 5 ) * 1 mm"
named bodies: "Circuit Board", "Pin Connector 3", "Pin Connector 5", "Pin Connector 1", "Pin Connector 7", "Pin Connector 4", "Pin Connector 6", "Pin Connector 2", "Pin Connector 8", "Pin 6", "Pin 2", "Pin 3", "Pin 8", "Pin 5", "Pin 1", "Pin 4", "Pin 7", "Back left LED", "Front Right LED", "Back right LED", "Front left LED", "Colour Sensor Holder", "Colour Sensor Matrix"
